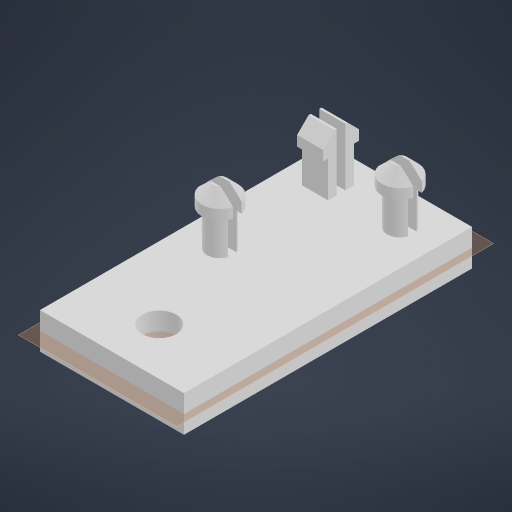
# Autodesk Inventor part: MirrorBaseplate
Saved by Autodesk Inventor 2024.1 (Build 281209000, 209)
## iProperties
Created: 2023-08-17
Part Number: MirrorBaseplate
Material: Generic
Document SubType Name: Modeling
Designer: Eleanor
Density: 1 g/cm^3
Appearance: Default
Author: Eleanor
Autodesk Inventor part; units mm, degrees
ref_plane "YZ Plane" through (0, 0, 0) normal (1, 0, 0) x (0, 1, 0)
ref_plane "XZ Plane" through (0, 0, 0) normal (0, 1, 0) x (-1, 0, 0)
ref_plane "XY Plane" through (0, 0, 0) normal (0, 0, 1) x (1, 0, 0)
sketch "Sketch1" plane through (0, 0, 0) normal (0, 1, 0) x (-1, 0, 0)
  line L0 (-6.35, 12.7) -> (-6.35, -12.7)
  line L1 (-6.35, -12.7) -> (6.35, -12.7)
  line L2 (6.35, -12.7) -> (6.35, 12.7)
  line L3 (6.35, 12.7) -> (-6.35, 12.7)
  line L4 (-6.35, 12.7) -> (6.35, -12.7) construction
  line L5 (-6.35, -12.7) -> (6.35, 12.7) construction
  line L6 (-6.35, 12.7) -> (19.05, 12.7) construction
  point P0 (0, 0)
  dimension "d0" = 25.4
  dimension "d1" = 90
  dimension "d2" = 12.7
  constraints: 14 end point, 2 midpoint, 2 parallel, 2 perpendicular, 1 horizontal, 1 vertical
  measures "d0" distance of L0.start L0.end
  measures "d1" angle of L0 L6
  measures "d2" distance of L1.end L0.end
extrude "Baseplate" add sketch "Sketch1" against normal blind 3.175
sketch "Sketch2" plane through (0, -3.175, 0) normal (0, -1, 0) x (1, 0, 0)
  circle A0 centre (3.175, -9.525) radius 1.143
  circle A1 centre (-3.175, 0) radius 1.143
  circle A2 centre (0, 8.5298) radius 1.5
  line L0 (-4.318, -8.382) -> (-2.032, -8.382)
  line L1 (-2.032, -8.382) -> (-2.032, -10.668)
  line L2 (-2.032, -10.668) -> (-4.318, -10.668)
  line L3 (-4.318, -10.668) -> (-4.318, -8.382)
  line L4 (-4.318, -8.382) -> (-2.032, -10.668) construction
  line L5 (-2.032, -8.382) -> (-4.318, -10.668) construction
  point P0 (0, 0)
  point P1 (-3.175, -9.525)
  dimension "d5" = 2.286
  dimension "d6" = 2.286
  dimension "d7" = 3
  dimension "d8" = 2.286
  constraints: 12 end point, 3 centre point, 2 midpoint, 2 parallel, 1 horizontal, 1 perpendicular
  measures "d5" diameter of A0
  measures "d6" diameter of A1
  measures "d7" diameter of A2
  measures "d8" distance of L1.end L2.end
extrude "BoltHole" cut sketch "Sketch2" against normal blind 3.175 contours A2
extrude "Extrusion3" add sketch "Sketch2" along normal blind 3.175 contours A0 | A1 | L0 L1 L2 L3
sketch "Sketch3" plane through (0, -6.35, 0) normal (0, -1, 0) x (1, 0, 0)
  line L0 (-2.032, -11.1125) -> (-4.318, -11.1125)
  line L1 (-4.318, -11.1125) -> (-4.318, -7.9375)
  line L2 (-4.318, -7.9375) -> (-2.032, -7.9375)
  line L3 (-2.032, -7.9375) -> (-2.032, -11.1125)
  line L4 (-2.032, -11.1125) -> (-4.318, -7.9375) construction
  line L5 (-4.318, -11.1125) -> (-2.032, -7.9375) construction
  circle A0 centre (-3.175, 0) radius 1.143 projected
  circle A1 centre (-3.175, 0) radius 1.5875
  circle A2 centre (3.175, -9.525) radius 1.5875
  point P0 (0, 0)
  point P1 (-3.175, -9.525)
  dimension "d13" = 2.286
  dimension "d14" = 3.175
  dimension "d15" = 3.175
  dimension "d16" = 3.175
  constraints: 12 end point, 2 centre point, 2 midpoint, 2 parallel, 1 coincident, 1 horizontal, 1 perpendicular
  measures "d13" distance of L1.end L2.end
  measures "d14" distance of L0.end L1.end
  measures "d15" diameter of A1
  measures "d16" diameter of A2
extrude "Extrusion4" add sketch "Sketch3" along normal blind 1.905 contours L0 L1 L2 L3 | A0 | A1 | A2
chamfer "Chamfer1" distance 1.016 angle 45 4 edges at (-4.7625, -8.255, 0) (1.5875, -8.255, -9.525) (-3.175, -8.255, -7.9375) (-3.175, -8.255, -11.1125)
sketch "Sketch4" plane through (0, -8.255, 0) normal (0, -1, 0) x (1, 0, 0)
  line L0 (5.202, -9.144) -> (1.148, -9.144)
  line L1 (1.148, -9.144) -> (1.148, -9.906)
  line L2 (1.148, -9.906) -> (5.202, -9.906)
  line L3 (5.202, -9.906) -> (5.202, -9.144)
  circle A0 centre (3.175, -9.525) radius 0.5715 projected
  line L4 (5.202, -9.144) -> (1.148, -9.906) construction
  line L5 (1.148, -9.144) -> (5.202, -9.906) construction
  line L6 (-0.7593, 0.381) -> (-5.5907, 0.381)
  line L7 (-5.5907, 0.381) -> (-5.5907, -0.381)
  line L8 (-5.5907, -0.381) -> (-0.7593, -0.381)
  line L9 (-0.7593, -0.381) -> (-0.7593, 0.381)
  line L10 (-0.7593, 0.381) -> (-5.5907, -0.381) construction
  line L11 (-5.5907, 0.381) -> (-0.7593, -0.381) construction
  line L12 (-5.5907, -9.906) -> (-0.7593, -9.906)
  line L13 (-0.7593, -9.906) -> (-0.7593, -9.144)
  line L14 (-0.7593, -9.144) -> (-5.5907, -9.144)
  line L15 (-5.5907, -9.144) -> (-5.5907, -9.906)
  line L16 (-5.5907, -9.906) -> (-0.7593, -9.144) construction
  line L17 (-0.7593, -9.906) -> (-5.5907, -9.144) construction
  point P0 (0, 0)
  point P1 (-3.175, 0)
  point P2 (-3.175, -9.525)
  dimension "d24" = 0.762
  dimension "d25" = 0.762
  constraints: 36 end point, 6 midpoint, 6 parallel, 3 horizontal, 3 perpendicular
  measures "d24" distance of L1.end L0.end
  measures "d25" distance of L7.end L6.end
extrude "Extrusion5" cut sketch "Sketch4" against normal blind 5.08 contours L3 L2 A0 L0 | A0 L2 L0 | A0 L2 L1 L0 | L9 L8 L7 L6 | L15 L14 L13 L12
ref_plane "Work Plane1" through (0, -1.5875, 0) normal (0, 1, 0) x (1, 0, 0)
mirror "Mirror1" about plane through (0, -1.5875, 0) normal (0, 1, 0) of "Extrusion3", "Extrusion4", "Chamfer1", "Extrusion5"
sketch "Sketch5" plane through (0, -3.175, 0) normal (0, -1, 0) x (1, 0, 0)
  line L0 (-6.35, 12.7) -> (-6.35, -12.7) projected
  line L1 (6.35, 12.7) -> (6.35, -12.7) projected
  line L2 (-6.35, -12.7) -> (6.35, -12.7)
  line L3 (6.35, -12.7) -> (6.35, 12.7)
  line L4 (6.35, 12.7) -> (-6.35, 12.7)
  line L5 (-6.35, 12.7) -> (-6.35, -12.7)
  point P0 (0, 0)
  constraints: 8 end point, 2 parallel, 1 horizontal, 1 perpendicular
extrude "Extrusion6" cut sketch "Sketch5" along normal blind 6.0325
body "Solid1"
